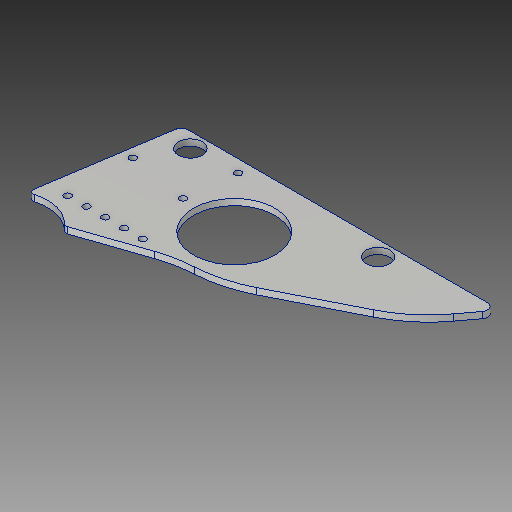
# Autodesk Inventor part: Flywheel Bracket 1
Saved by Autodesk Inventor 2019.4 (Build 234330000, 330)
## iProperties
Created: 2020-01-06
Part Number: Flywheel Bracket 1
Material: Aluminum 6061
Document SubType Name: Modeling
Designer: admin
Density: 2.7 g/cm^3
Appearance: Aluminum - Flat
Author: admin
Autodesk Inventor part; units mm, degrees
ref_plane "YZ Plane" through (0, 0, 0) normal (1, 0, 0) x (0, 1, 0)
ref_plane "XZ Plane" through (0, 0, 0) normal (0, 1, 0) x (-1, 0, 0)
ref_plane "XY Plane" through (0, 0, 0) normal (0, 0, 1) x (1, 0, 0)
sketch "Sketch1" plane through (0, 0, 0) normal (0, 1, 0) x (-1, 0, 0)
  circle A0 centre (0, 0) radius 9.5
  circle A1 centre (75, 40) radius 9.5 construction
  line L0 (75, 40) -> (0, 0) construction
  line L1 (168.5523, -12) -> (-85.507, -12)
  line L2 (-85.507, -12) -> (-55.507, 28)
  line L3 (-55.507, 28) -> (48.5523, 80.4961)
  line L4 (48.5523, 80.4961) -> (78.5523, 80.4961)
  circle A2 centre (0, 0) radius 40 construction
  circle A3 centre (150, 0) radius 9.5
  line L5 (168.5523, -12) -> (188.5523, 118)
  line L6 (188.5523, 118) -> (78.5523, 80.4961)
  arc A4 (190.616, -6.9524) -> (186.8364, 18.756) centre (149.966, 0.2035) ccw
  circle A5 centre (75, 40) radius 14.0208 construction
  circle A6 centre (75, 40) radius 32.5
  dimension "d0" = 19
  dimension "d1" = 19
  dimension "d2" = 85
  dimension "d4" = 80
  dimension "d5" = 12
  dimension "d6" = 50
  dimension "d12" = 19
  dimension "d18" = 20
  dimension "d25" = 30
  dimension "d26" = 30
  dimension "d27" = 40
  dimension "d28" = 130
  dimension "d29" = 110
  dimension "d34" = 150
  dimension "d35" = 0
  dimension "d36" = 65
  constraints: 14 end point, 6 centre point, 4 coincident, 2 point on circle, 1 horizontal, 1 parallel, 3 other
  measures "d0" diameter of A0
  measures "d1" diameter of A1
  measures "d2" distance of L0.start L0.end
  measures "d4" diameter of A2
  measures "d5" distance from line of L0.end L1
  measures "d6" distance from line of A2.centre L3
  measures "d12" diameter of A3
  measures "d18" horizontal distance of L1.start L5.end
  measures "d25" distance of L4.end L3.end
  measures "d26" horizontal distance of L1.end L2.end
  measures "d27" vertical distance of L1.end L2.end
  measures "d28" vertical distance of L1.start L5.end
  measures "d29" horizontal distance of L5.end L4.end
  measures "d34" distance of L0.end A3.centre
  measures "d35" vertical distance of A3.centre L0.end
  measures "d36" diameter of A6
extrude "Extrusion1" add sketch "Sketch1" along normal blind 5
fillet "Fillet1" radius 5 2 edges at (85.507, 2.5, -12) (-168.5523, 2.5, -12)
fillet "Fillet2" radius 100 2 edges at (55.507, 2.5, 28) (-48.5523, 2.5, 80.4961)
fillet "Fillet3" radius 10 1 edges at (-188.5523, 2.5, 118)
fillet "Fillet4" radius 100 1 edges at (-78.5523, 2.5, 80.4961)
sketch "Sketch2" plane through (0, 5, 0) normal (0, 1, 0) x (1, 0, 0)
  circle A0 centre (-106.4222, -81.641) radius 2.75 projected
  circle A1 centre (-121.4222, -81.641) radius 2.75 projected
  circle A2 centre (-136.4222, -81.641) radius 2.75 projected
  circle A3 centre (-151.4222, -81.641) radius 2.75 projected
  circle A4 centre (-166.4222, -81.641) radius 2.75 projected
  point P0 (0, 0)
extrude "Extrusion2" cut sketch "Sketch2" against normal through all
sketch "Sketch3" plane through (0, 5, 0) normal (0, 1, 0) x (1, 0, 0)
  circle A0 centre (-166.6168, -29.3999) radius 2.75 projected
  circle A1 centre (-118.5529, -37.5005) radius 2.75 projected
  circle A2 centre (-114.0019, 2.0311) radius 2.75 projected
  point P0 (0, 0)
extrude "Extrusion3" cut sketch "Sketch3" against normal through all
sketch "Sketch4" plane through (0, 5, 0) normal (0, 1, 0) x (1, 0, 0)
  circle A0 centre (-171.3333, -125.7026) radius 30.877 projected
  circle A1 centre (-171.3333, -125.7026) radius 9.525 projected
  circle A2 centre (-188.1943, -144.6991) radius 2.0193 projected
  circle A3 centre (-154.4723, -106.7061) radius 2.0193 projected
  circle A4 centre (-171.3333, -125.7026) radius 32.877
  point P0 (0, 0)
  dimension "d30" = 2
  constraints: 1 centre point
  measures "d30" radial gap between concentric circles of A0 A4
extrude "Extrusion4" cut sketch "Sketch4" against normal through all contours A0 | A2 | A3 | A4
fillet "Fillet5" radius 3 2 edges at (-146.8352, 2.5, 103.7768) (-185.1475, 2.5, 95.8686)
body "Solid1"
